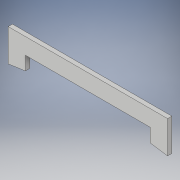
# Autodesk Inventor part: Skateboard Electronics Box
Saved by Autodesk Inventor 2017.3 (Build 213256000, 256)
## iProperties
Created: 2019-01-08
Part Number: Skateboard Electronics Box
Material: Generic
Document SubType Name: Modeling
Designer: LSabe
Density: 1 g/cm^3
Appearance: Default
Author: LSabe
Autodesk Inventor part; units mm, degrees
ref_plane "YZ Plane" through (0, 0, 0) normal (1, 0, 0) x (0, 1, 0)
ref_plane "XZ Plane" through (0, 0, 0) normal (0, 1, 0) x (-1, 0, 0)
ref_plane "XY Plane" through (0, 0, 0) normal (0, 0, 1) x (1, 0, 0)
sketch "Sketch1" plane through (0, 0, 0) normal (0, 0, 1) x (1, 0, 0)
  line L0 (114.2744, 165.7819) -> (114.2744, 213.4069)
  line L1 (114.2744, 213.4069) -> (349.2244, 213.4069)
  line L2 (114.2744, 213.4069) -> (349.2244, 213.4069) construction
  line L3 (349.2244, 213.4069) -> (349.2244, 165.7819)
  line L4 (139.6744, 189.5944) -> (139.6744, 169.4704)
  line L5 (139.6744, 189.5944) -> (231.7494, 189.5944)
  line L6 (139.6744, 189.5944) -> (231.7494, 189.5944) construction
  line L7 (323.8244, 189.5944) -> (323.8244, 169.4704)
  line L8 (323.8244, 189.5944) -> (231.7494, 189.5944)
  line L9 (323.8244, 189.5944) -> (231.7494, 189.5944) construction
  line L10 (231.7494, 189.5944) -> (231.7494, 175.3069)
  arc A0 (349.2244, 165.7819) -> (323.8244, 169.4704) centre (231.7494, -553.8848) ccw
  arc A1 (139.6744, 169.4704) -> (114.2744, 165.7819) centre (231.7494, -553.8848) ccw
  constraints: 22 end point, 4 point on circle, 2 centre point, 2 collinear, 2 horizontal, 1 perpendicular, 1 vertical
extrude "Extrusion1" add sketch "Sketch1" along normal blind 6.35
body "Solid1"
